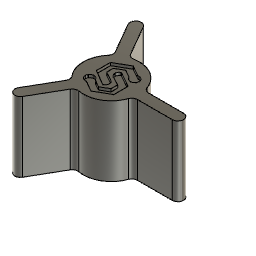
Rotary Cap (Autodesk Fusion 360 design; units mm, degrees)
Autodesk Fusion 360 part; units mm, degrees
note: some values were not read from the file. Set by a fixed rule: which sketch regions a step uses.
sketch "Sketch1" plane through (0, 0, 0) normal (0, 0, 1) x (1, 0, 0)
  circle A0 centre (0, 0) radius 3.15
  line L0 (0, 0) -> (-3.15, 0) construction
  line L1 (-3.15, 0) -> (-3.15, 4) construction
  line L2 (1.4, 2.8218) -> (1.4, -2.8218)
  line L3 (0, 0) -> (7.7021, 0) construction
  line L4 (12.899, 1) -> (4.899, 1)
  line L5 (4.899, -1) -> (12.8981, -1)
  line L6 (12.8981, -1) -> (12.899, 1)
  line L7 (12.899, 1) -> (7.0944, 0) construction
  line L8 (7.0944, 0) -> (12.8981, -1) construction
  arc A1 (4.899, 1) -> (4.899, -1) centre (0, 0) ccw
  line L9 (-7.3155, 10.6708) -> (-3.3155, 3.7426)
  line L10 (-1.5835, 4.7426) -> (-5.583, 11.6701)
  line L11 (-5.583, 11.6701) -> (-7.3155, 10.6708)
  line L12 (-5.5835, -11.6708) -> (-1.5835, -4.7426)
  line L13 (-3.3155, -3.7426) -> (-7.3151, -10.6701)
  line L14 (-7.3151, -10.6701) -> (-5.5835, -11.6708)
  dimension "d1" = 6.3
  dimension "d2" = 4.55
  dimension "d3" = 10
  dimension "d12" = 8
  dimension "d14" = 360
  dimension "d15" = 2
  dimension "d16" = 1
  constraint coincident A0.centre L0.start
  constraint coincident A0 L0.end
  constraint horizontal L0
  constraint tangent A0 L1
  constraint coincident A0 L2.start
  constraint coincident A0 L2.end
  constraint vertical L2
  constraint perpendicular L2 L3
  constraint horizontal L4
  constraint parallel L4 L5
  constraint coincident L3 L7.end
  measures "d1" diameter of A0
  measures "d2" distance of L1 L2
  measures "d3" diameter of A1
  measures "d12" distance of L6 L4.end
  measures "d15" distance of L4 L5
  measures "d16" distance of L3 L4
extrude "Extrude1" add sketch "Sketch1" along normal blind 12.5 contours A0 L2 | L4 L5 L6 A1 | A1 L9 L10 L11 | A1 L12 L13 L14 picked at (2.2591, -0.5149)
sketch "Sketch2" plane through (0, 0, 12.5) normal (0, 0, 1) x (-1, 0, 0)
  arc A0 (-1.4, -2.8218) -> (-1.4, 2.8218) centre (0, 0) ccw
  line L0 (-1.4, -2.8218) -> (-1.4, 2.8218)
  arc A1 (1.5835, 4.7426) -> (-4.899, 1) centre (0, 0) ccw
  line L1 (-4.899, 1) -> (-12.8981, 1)
  line L2 (-12.8981, 1) -> (-12.899, -1)
  line L3 (-12.899, -1) -> (-4.899, -1)
  circle A2 centre (0, 0) radius 3.15
  line L4 (7.3151, 10.6701) -> (5.5835, 11.6708)
  line L5 (5.5835, 11.6708) -> (1.5835, 4.7426)
  arc A3 (-4.899, -1) -> (1.5835, -4.7426) centre (0, 0) ccw
  line L6 (1.5835, -4.7426) -> (5.583, -11.6701)
  line L7 (5.583, -11.6701) -> (7.3155, -10.6708)
  line L8 (7.3155, -10.6708) -> (3.3155, -3.7426)
  arc A4 (3.3155, -3.7426) -> (3.3155, 3.7426) centre (0, 0) ccw
  line L9 (3.3155, 3.7426) -> (7.3151, 10.6701)
  constraint coincident A0.centre A1.centre
  constraint coincident A0.start A2
extrude "Extrude2" add sketch "Sketch2" against normal blind 2 contours A0 L0 A2
fillet "Fillet1" radius 1 12 edges at (4.899, -1, 6.25) (12.8981, -1, 6.25) (12.899, 1, 6.25) (4.899, 1, 6.25) (-1.5835, -4.7426, 6.25) (-3.3155, -3.7426, 6.25) (-3.3155, 3.7426, 6.25) (-1.5835, 4.7426, 6.25) (-5.5835, -11.6708, 6.25) (-7.3151, -10.6701, 6.25) (-7.3155, 10.6708, 6.25) (-5.583, 11.6701, 6.25)
sketch "Sketch3" plane through (0, 0, 12.5) normal (0, 0, 1) x (-1, 0, 0)
  arc A0 (-11.8986, 1) -> (-11.8986, -1) centre (-11.8986, 0) ccw
  line L0 (-11.8986, -1) -> (-5.6569, -1)
  arc A1 (-4.714, -1.6667) -> (-5.6569, -1) centre (-5.6569, -2) ccw
  arc A2 (-4.714, -1.6667) -> (0.9136, -4.9158) centre (0, 0) ccw
  arc A3 (-5.6569, 1) -> (-4.714, 1.6667) centre (-5.6569, 2) ccw
  line L1 (-5.6569, 1) -> (-11.8986, 1)
  spline S0 degree 3 poles (-6.2098, 2.4164) (-5.9078, 2.4164) (-5.6092, 2.3629) (-5.3142, 2.2561) knots 0 0 0 0 1 1 1 1
  spline S1 degree 3 poles (-5.3142, 2.2561) (-5.019, 2.1491) (-4.7505, 1.9819) (-4.509, 1.7542) knots 0 0 0 0 1 1 1 1
  line L2 (-4.509, 1.7542) -> (-5.0946, 1.0362)
  spline S2 degree 3 poles (-5.0946, 1.0362) (-5.2572, 1.171) (-5.4407, 1.2743) (-5.6453, 1.3463) knots 0 0 0 0 1 1 1 1
  spline S3 degree 3 poles (-5.6453, 1.3463) (-5.8497, 1.4185) (-6.0471, 1.4544) (-6.2377, 1.4544) knots 0 0 0 0 1 1 1 1
  spline S4 degree 3 poles (-6.2377, 1.4544) (-6.433, 1.4544) (-6.5781, 1.4219) (-6.6735, 1.3569) knots 0 0 0 0 1 1 1 1
  spline S5 degree 3 poles (-6.6735, 1.3569) (-6.7686, 1.2918) (-6.8164, 1.1989) (-6.8164, 1.078) knots 0 0 0 0 1 1 1 1
  spline S6 degree 3 poles (-6.8164, 1.078) (-6.8164, 0.9897) (-6.7896, 0.9201) (-6.7362, 0.8688) knots 0 0 0 0 1 1 1 1
  spline S7 degree 3 poles (-6.7362, 0.8688) (-6.6827, 0.8178) (-6.6096, 0.7713) (-6.5165, 0.7295) knots 0 0 0 0 1 1 1 1
  spline S8 degree 3 poles (-6.5165, 0.7295) (-6.4236, 0.6876) (-6.3121, 0.6413) (-6.182, 0.59) knots 0 0 0 0 1 1 1 1
  line L3 (-6.182, 0.59) -> (-5.6034, 0.3461)
  spline S9 degree 3 poles (-5.6034, 0.3461) (-5.4407, 0.281) (-5.2898, 0.1927) (-5.1503, 0.0812) knots 0 0 0 0 1 1 1 1
  spline S10 degree 3 poles (-5.1503, 0.0812) (-5.0109, -0.0304) (-4.8982, -0.1686) (-4.8122, -0.3336) knots 0 0 0 0 1 1 1 1
  spline S11 degree 3 poles (-4.8122, -0.3336) (-4.7262, -0.4985) (-4.6833, -0.6902) (-4.6833, -0.9087) knots 0 0 0 0 1 1 1 1
  spline S12 degree 3 poles (-4.6833, -0.9087) (-4.6833, -1.1642) (-4.7541, -1.3954) (-4.896, -1.6022) knots 0 0 0 0 1 1 1 1
  spline S13 degree 3 poles (-4.896, -1.6022) (-5.0376, -1.809) (-5.2327, -1.9751) (-5.4814, -2.1007) knots 0 0 0 0 1 1 1 1
  spline S14 degree 3 poles (-5.4814, -2.1007) (-5.7299, -2.2261) (-6.0169, -2.2889) (-6.3423, -2.2889) knots 0 0 0 0 1 1 1 1
  spline S15 degree 3 poles (-6.3423, -2.2889) (-6.6164, -2.2889) (-6.8826, -2.24) (-7.1404, -2.1425) knots 0 0 0 0 1 1 1 1
  spline S16 degree 3 poles (-7.1404, -2.1425) (-7.3984, -2.0449) (-7.625, -1.9032) (-7.8201, -1.7173) knots 0 0 0 0 1 1 1 1
  line L4 (-7.8201, -1.7173) -> (-7.2416, -0.9923)
  spline S17 degree 3 poles (-7.2416, -0.9923) (-7.0882, -1.1039) (-6.936, -1.1875) (-6.785, -1.2432) knots 0 0 0 0 1 1 1 1
  spline S18 degree 3 poles (-6.785, -1.2432) (-6.6339, -1.299) (-6.4863, -1.3269) (-6.3423, -1.3269) knots 0 0 0 0 1 1 1 1
  spline S19 degree 3 poles (-6.3423, -1.3269) (-6.1797, -1.3269) (-6.0506, -1.2966) (-5.9555, -1.2363) knots 0 0 0 0 1 1 1 1
  spline S20 degree 3 poles (-5.9555, -1.2363) (-5.8601, -1.1758) (-5.8125, -1.0875) (-5.8125, -0.9714) knots 0 0 0 0 1 1 1 1
  spline S21 degree 3 poles (-5.8125, -0.9714) (-5.8125, -0.8924) (-5.8404, -0.825) (-5.8962, -0.7692) knots 0 0 0 0 1 1 1 1
  spline S22 degree 3 poles (-5.8962, -0.7692) (-5.952, -0.7135) (-6.0321, -0.6647) (-6.1367, -0.6229) knots 0 0 0 0 1 1 1 1
  spline S23 degree 3 poles (-6.1367, -0.6229) (-6.2413, -0.581) (-6.3608, -0.5323) (-6.4957, -0.4764) knots 0 0 0 0 1 1 1 1
  line L5 (-6.4957, -0.4764) -> (-7.0602, -0.2534)
  spline S24 degree 3 poles (-7.0602, -0.2534) (-7.2461, -0.179) (-7.4053, -0.0849) (-7.5378, 0.0289) knots 0 0 0 0 1 1 1 1
  spline S25 degree 3 poles (-7.5378, 0.0289) (-7.6702, 0.1428) (-7.7723, 0.2776) (-7.8445, 0.4331) knots 0 0 0 0 1 1 1 1
  spline S26 degree 3 poles (-7.8445, 0.4331) (-7.9165, 0.589) (-7.9526, 0.7737) (-7.9526, 0.9873) knots 0 0 0 0 1 1 1 1
  spline S27 degree 3 poles (-7.9526, 0.9873) (-7.9526, 1.243) (-7.8852, 1.4788) (-7.7504, 1.6949) knots 0 0 0 0 1 1 1 1
  spline S28 degree 3 poles (-7.7504, 1.6949) (-7.6156, 1.911) (-7.4181, 2.0853) (-7.1579, 2.2178) knots 0 0 0 0 1 1 1 1
  spline S29 degree 3 poles (-7.1579, 2.2178) (-6.8975, 2.3502) (-6.5816, 2.4164) (-6.2098, 2.4164) knots 0 0 0 0 1 1 1 1
  spline S30 degree 3 poles (-10.3713, 1.4544) (-10.5666, 1.4544) (-10.735, 1.3976) (-10.8767, 1.2836) knots 0 0 0 0 1 1 1 1
  spline S31 degree 3 poles (-10.8767, 1.2836) (-11.0184, 1.1698) (-11.1265, 1.0072) (-11.2009, 0.7957) knots 0 0 0 0 1 1 1 1
  spline S32 degree 3 poles (-11.2009, 0.7957) (-11.2752, 0.5842) (-11.3124, 0.3345) (-11.3124, 0.0463) knots 0 0 0 0 1 1 1 1
  spline S33 degree 3 poles (-11.3124, 0.0463) (-11.3124, -0.2465) (-11.2752, -0.4939) (-11.2009, -0.6961) knots 0 0 0 0 1 1 1 1
  spline S34 degree 3 poles (-11.2009, -0.6961) (-11.1265, -0.8982) (-11.0184, -1.0539) (-10.8767, -1.1632) knots 0 0 0 0 1 1 1 1
  spline S35 degree 3 poles (-10.8767, -1.1632) (-10.735, -1.2722) (-10.5666, -1.3269) (-10.3713, -1.3269) knots 0 0 0 0 1 1 1 1
  spline S36 degree 3 poles (-10.3713, -1.3269) (-10.1762, -1.3269) (-10.0077, -1.2722) (-9.8659, -1.1632) knots 0 0 0 0 1 1 1 1
  spline S37 degree 3 poles (-9.8659, -1.1632) (-9.7242, -1.0539) (-9.6162, -0.8982) (-9.5419, -0.6961) knots 0 0 0 0 1 1 1 1
  spline S38 degree 3 poles (-9.5419, -0.6961) (-9.4675, -0.4939) (-9.4303, -0.2465) (-9.4303, 0.0463) knots 0 0 0 0 1 1 1 1
  spline S39 degree 3 poles (-9.4303, 0.0463) (-9.4303, 0.3345) (-9.4675, 0.5842) (-9.5419, 0.7957) knots 0 0 0 0 1 1 1 1
  spline S40 degree 3 poles (-9.5419, 0.7957) (-9.6162, 1.0072) (-9.7242, 1.1698) (-9.8659, 1.2836) knots 0 0 0 0 1 1 1 1
  spline S41 degree 3 poles (-9.8659, 1.2836) (-10.0077, 1.3976) (-10.1762, 1.4544) (-10.3713, 1.4544) knots 0 0 0 0 1 1 1 1
  spline S42 degree 3 poles (-10.3713, 2.4164) (-9.9577, 2.4164) (-9.5941, 2.3223) (-9.2804, 2.1341) knots 0 0 0 0 1 1 1 1
  spline S43 degree 3 poles (-9.2804, 2.1341) (-8.9668, 1.9458) (-8.7228, 1.674) (-8.5486, 1.3185) knots 0 0 0 0 1 1 1 1
  spline S44 degree 3 poles (-8.5486, 1.3185) (-8.3743, 0.963) (-8.287, 0.5389) (-8.287, 0.0463) knots 0 0 0 0 1 1 1 1
  spline S45 degree 3 poles (-8.287, 0.0463) (-8.287, -0.451) (-8.3743, -0.8727) (-8.5486, -1.2188) knots 0 0 0 0 1 1 1 1
  spline S46 degree 3 poles (-8.5486, -1.2188) (-8.7228, -1.565) (-8.9668, -1.8299) (-9.2804, -2.0135) knots 0 0 0 0 1 1 1 1
  spline S47 degree 3 poles (-9.2804, -2.0135) (-9.5941, -2.1971) (-9.9577, -2.2889) (-10.3713, -2.2889) knots 0 0 0 0 1 1 1 1
  spline S48 degree 3 poles (-10.3713, -2.2889) (-10.7849, -2.2889) (-11.1486, -2.1971) (-11.4623, -2.0135) knots 0 0 0 0 1 1 1 1
  spline S49 degree 3 poles (-11.4623, -2.0135) (-11.7759, -1.8299) (-12.0199, -1.565) (-12.1943, -1.2188) knots 0 0 0 0 1 1 1 1
  spline S50 degree 3 poles (-12.1943, -1.2188) (-12.3685, -0.8727) (-12.4556, -0.451) (-12.4556, 0.0463) knots 0 0 0 0 1 1 1 1
  spline S51 degree 3 poles (-12.4556, 0.0463) (-12.4556, 0.5389) (-12.3685, 0.963) (-12.1943, 1.3185) knots 0 0 0 0 1 1 1 1
  spline S52 degree 3 poles (-12.1943, 1.3185) (-12.0199, 1.674) (-11.7759, 1.9458) (-11.4623, 2.1341) knots 0 0 0 0 1 1 1 1
  spline S53 degree 3 poles (-11.4623, 2.1341) (-11.1486, 2.3223) (-10.7849, 2.4164) (-10.3713, 2.4164) knots 0 0 0 0 1 1 1 1
  line L6 (-17.4953, 1.4404) -> (-17.6278, 1.4404)
  spline S54 degree 3 poles (-17.6278, 1.4404) (-17.8647, 1.4404) (-18.0763, 1.3986) (-18.2621, 1.315) knots 0 0 0 0 1 1 1 1
  spline S55 degree 3 poles (-18.2621, 1.315) (-18.448, 1.2314) (-18.5943, 1.0885) (-18.7013, 0.8862) knots 0 0 0 0 1 1 1 1
  spline S56 degree 3 poles (-18.7013, 0.8862) (-18.8081, 0.6841) (-18.8616, 0.4043) (-18.8616, 0.0462) knots 0 0 0 0 1 1 1 1
  spline S57 degree 3 poles (-18.8616, 0.0462) (-18.8616, -0.3115) (-18.8081, -0.588) (-18.7013, -0.7832) knots 0 0 0 0 1 1 1 1
  spline S58 degree 3 poles (-18.7013, -0.7832) (-18.5943, -0.9783) (-18.448, -1.1154) (-18.2621, -1.1944) knots 0 0 0 0 1 1 1 1
  spline S59 degree 3 poles (-18.2621, -1.1944) (-18.0763, -1.2735) (-17.8647, -1.313) (-17.6278, -1.313) knots 0 0 0 0 1 1 1 1
  line L7 (-17.6278, -1.313) -> (-17.4953, -1.313)
  line L8 (-17.4953, -1.313) -> (-17.4953, 1.4404)
  line L9 (-16.38, 2.3327) -> (-16.38, -2.2052)
  line L10 (-16.38, -2.2052) -> (-17.6975, -2.2052)
  spline S60 degree 3 poles (-17.6975, -2.2052) (-18.1576, -2.2052) (-18.5607, -2.1274) (-18.907, -1.9718) knots 0 0 0 0 1 1 1 1
  spline S61 degree 3 poles (-18.907, -1.9718) (-19.253, -1.816) (-19.5214, -1.5732) (-19.7121, -1.2432) knots 0 0 0 0 1 1 1 1
  spline S62 degree 3 poles (-19.7121, -1.2432) (-19.9025, -0.9132) (-19.9978, -0.4835) (-19.9978, 0.0462) knots 0 0 0 0 1 1 1 1
  spline S63 degree 3 poles (-19.9978, 0.0462) (-19.9978, 0.5715) (-19.9025, 1.0026) (-19.7121, 1.3394) knots 0 0 0 0 1 1 1 1
  spline S64 degree 3 poles (-19.7121, 1.3394) (-19.5214, 1.6764) (-19.2578, 1.9261) (-18.9209, 2.0887) knots 0 0 0 0 1 1 1 1
  spline S65 degree 3 poles (-18.9209, 2.0887) (-18.5839, 2.2514) (-18.197, 2.3327) (-17.7602, 2.3327) knots 0 0 0 0 1 1 1 1
  line L11 (-17.7602, 2.3327) -> (-16.38, 2.3327)
  line L12 (-20.5074, 2.3327) -> (-20.5074, -2.2052)
  line L13 (-20.5074, -2.2052) -> (-23.4002, -2.2052)
  line L14 (-23.4002, -2.2052) -> (-23.4002, -1.2711)
  line L15 (-23.4002, -1.2711) -> (-21.6227, -1.2711)
  line L16 (-21.6227, -1.2711) -> (-21.6227, -0.4625)
  line L17 (-21.6227, -0.4625) -> (-23.1354, -0.4625)
  line L18 (-23.1354, -0.4625) -> (-23.1354, 0.4715)
  line L19 (-23.1354, 0.4715) -> (-21.6227, 0.4715)
  line L20 (-21.6227, 0.4715) -> (-21.6227, 1.3986)
  line L21 (-21.6227, 1.3986) -> (-23.47, 1.3986)
  line L22 (-23.47, 1.3986) -> (-23.47, 2.3327)
  line L23 (-23.47, 2.3327) -> (-20.5074, 2.3327)
  line L24 (-25.1917, -1.32) -> (-25.6727, -1.32)
  spline S66 degree 3 poles (-25.6727, -1.32) (-25.9236, -1.32) (-26.1152, -1.2804) (-26.2477, -1.2015) knots 0 0 0 0 1 1 1 1
  spline S67 degree 3 poles (-26.2477, -1.2015) (-26.3801, -1.1224) (-26.4464, -0.9759) (-26.4464, -0.7623) knots 0 0 0 0 1 1 1 1
  spline S68 degree 3 poles (-26.4464, -0.7623) (-26.4464, -0.5531) (-26.3801, -0.3951) (-26.2477, -0.2882) knots 0 0 0 0 1 1 1 1
  spline S69 degree 3 poles (-26.2477, -0.2882) (-26.1152, -0.1813) (-25.9236, -0.128) (-25.6727, -0.128) knots 0 0 0 0 1 1 1 1
  line L25 (-25.6727, -0.128) -> (-25.1917, -0.128)
  line L26 (-25.1917, -0.128) -> (-25.1917, -1.32)
  line L27 (-27.7709, 2.3327) -> (-26.7633, 0.5394)
  spline S70 degree 3 poles (-26.7633, 0.5394) (-26.9762, 0.4339) (-27.1545, 0.2898) (-27.2934, 0.1021) knots 0 0 0 0 1 1 1 1
  spline S71 degree 3 poles (-27.2934, 0.1021) (-27.4583, -0.121) (-27.5409, -0.4091) (-27.5409, -0.7623) knots 0 0 0 0 1 1 1 1
  spline S72 degree 3 poles (-27.5409, -0.7623) (-27.5409, -1.134) (-27.4583, -1.4246) (-27.2934, -1.6336) knots 0 0 0 0 1 1 1 1
  spline S73 degree 3 poles (-27.2934, -1.6336) (-27.1283, -1.8427) (-26.9111, -1.9902) (-26.6416, -2.0763) knots 0 0 0 0 1 1 1 1
  spline S74 degree 3 poles (-26.6416, -2.0763) (-26.372, -2.1623) (-26.0769, -2.2052) (-25.7564, -2.2052) knots 0 0 0 0 1 1 1 1
  line L28 (-25.7564, -2.2052) -> (-24.0764, -2.2052)
  line L29 (-24.0764, -2.2052) -> (-24.0764, 2.3327)
  line L30 (-24.0764, 2.3327) -> (-25.1917, 2.3327)
  line L31 (-25.1917, 2.3327) -> (-25.1917, 0.7574)
  line L32 (-25.1917, 0.7574) -> (-25.7071, 0.7574)
  line L33 (-25.7071, 0.7574) -> (-26.5301, 2.3327)
  line L34 (-26.5301, 2.3327) -> (-27.7709, 2.3327)
  line L35 (-28.2029, 2.3327) -> (-28.2029, -2.2052)
  line L36 (-28.2029, -2.2052) -> (-31.0958, -2.2052)
  line L37 (-31.0958, -2.2052) -> (-31.0958, -1.2711)
  line L38 (-31.0958, -1.2711) -> (-29.3182, -1.2711)
  line L39 (-29.3182, -1.2711) -> (-29.3182, -0.4625)
  line L40 (-29.3182, -0.4625) -> (-30.8309, -0.4625)
  line L41 (-30.8309, -0.4625) -> (-30.8309, 0.4715)
  line L42 (-30.8309, 0.4715) -> (-29.3182, 0.4715)
  line L43 (-29.3182, 0.4715) -> (-29.3182, 1.3986)
  line L44 (-29.3182, 1.3986) -> (-31.1655, 1.3986)
  line L45 (-31.1655, 1.3986) -> (-31.1655, 2.3327)
  line L46 (-31.1655, 2.3327) -> (-28.2029, 2.3327)
  line L47 (-32.8176, 1.4404) -> (-32.95, 1.4404)
  spline S75 degree 3 poles (-32.95, 1.4404) (-33.187, 1.4404) (-33.3985, 1.3986) (-33.5843, 1.315) knots 0 0 0 0 1 1 1 1
  spline S76 degree 3 poles (-33.5843, 1.315) (-33.7702, 1.2314) (-33.9166, 1.0885) (-34.0235, 0.8862) knots 0 0 0 0 1 1 1 1
  spline S77 degree 3 poles (-34.0235, 0.8862) (-34.1303, 0.6841) (-34.1838, 0.4043) (-34.1838, 0.0462) knots 0 0 0 0 1 1 1 1
  spline S78 degree 3 poles (-34.1838, 0.0462) (-34.1838, -0.3115) (-34.1303, -0.588) (-34.0235, -0.7832) knots 0 0 0 0 1 1 1 1
  spline S79 degree 3 poles (-34.0235, -0.7832) (-33.9166, -0.9783) (-33.7702, -1.1154) (-33.5843, -1.1944) knots 0 0 0 0 1 1 1 1
  spline S80 degree 3 poles (-33.5843, -1.1944) (-33.3985, -1.2735) (-33.187, -1.313) (-32.95, -1.313) knots 0 0 0 0 1 1 1 1
  line L48 (-32.95, -1.313) -> (-32.8176, -1.313)
  line L49 (-32.8176, -1.313) -> (-32.8176, 1.4404)
  line L50 (-31.7023, 2.3327) -> (-31.7023, -2.2052)
  line L51 (-31.7023, -2.2052) -> (-33.0197, -2.2052)
  spline S81 degree 3 poles (-33.0197, -2.2052) (-33.4798, -2.2052) (-33.8829, -2.1274) (-34.2292, -1.9718) knots 0 0 0 0 1 1 1 1
  spline S82 degree 3 poles (-34.2292, -1.9718) (-34.5753, -1.816) (-34.8436, -1.5732) (-35.0343, -1.2432) knots 0 0 0 0 1 1 1 1
  spline S83 degree 3 poles (-35.0343, -1.2432) (-35.2248, -0.9132) (-35.32, -0.4835) (-35.32, 0.0462) knots 0 0 0 0 1 1 1 1
  spline S84 degree 3 poles (-35.32, 0.0462) (-35.32, 0.5715) (-35.2248, 1.0026) (-35.0343, 1.3394) knots 0 0 0 0 1 1 1 1
  spline S85 degree 3 poles (-35.0343, 1.3394) (-34.8436, 1.6764) (-34.5801, 1.9261) (-34.2431, 2.0887) knots 0 0 0 0 1 1 1 1
  spline S86 degree 3 poles (-34.2431, 2.0887) (-33.9061, 2.2514) (-33.5193, 2.3327) (-33.0825, 2.3327) knots 0 0 0 0 1 1 1 1
  line L52 (-33.0825, 2.3327) -> (-31.7023, 2.3327)
  line L53 (-14.6781, 1.2454) -> (-14.052, 0.6192)
  line L54 (-14.052, 0.6192) -> (-14.052, -2.2052)
  line L55 (-14.052, -2.2052) -> (-12.9366, -2.2052)
  line L56 (-12.9366, -2.2052) -> (-12.9366, 1.1617)
  line L57 (-12.9366, 1.1617) -> (-14.0947, 2.3197)
  line L58 (-14.0947, 2.3197) -> (-15.8425, 2.3197)
  line L59 (-15.8425, 2.3197) -> (-15.8425, 1.2454)
  line L60 (-15.8425, 1.2454) -> (-14.6781, 1.2454)
  line L61 (-2.2394, -2.7135) -> (-2.2375, -2.7135)
  spline S87 degree 3 poles (-2.2375, -2.7135) (-2.0945, -2.7132) (-1.9536, -2.7479) (-1.8297, -2.8194) knots 0 0 0 0 1 1 1 1
  line L62 (-1.8297, -2.8194) -> (-0.1005, -3.8178)
  line L63 (-0.1005, -3.8178) -> (2.4914, -2.3226)
  line L64 (2.4914, -2.3226) -> (2.4914, 0.1947)
  line L65 (2.4914, 0.1947) -> (-0.234, 1.7682)
  line L66 (-0.234, 1.7682) -> (-0.2972, 1.7352)
  spline S88 degree 3 poles (-0.2972, 1.7352) (-0.5334, 1.613) (-0.7079, 1.3532) (-0.7117, 1.0874) knots 0 0 0 0 1 1 1 1
  spline S89 degree 3 poles (-0.7117, 1.0874) (-0.7155, 0.8215) (-0.5476, 0.5233) (-0.3152, 0.3946) knots 0 0 0 0 1 1 1 1
  line L67 (-0.3152, 0.3946) -> (1.3304, -0.4892)
  line L68 (1.3304, -0.4892) -> (1.3304, -1.6688)
  line L69 (1.3304, -1.6688) -> (-0.0948, -2.4992)
  line L70 (-0.0948, -2.4992) -> (-1.2895, -1.8007)
  spline S90 degree 3 poles (-1.2895, -1.8007) (-1.4025, -1.7347) (-1.4943, -1.639) (-1.5608, -1.5262) knots 0 0 0 0 1 1 1 1
  spline S91 degree 3 poles (-1.5608, -1.5262) (-1.6978, -1.2941) (-1.9504, -1.1383) (-2.2394, -1.1383) knots 0 0 0 0 1 1 1 1
  spline S92 degree 3 poles (-2.2394, -1.1383) (-2.5025, -1.1383) (-2.7353, -1.2674) (-2.8784, -1.4657) knots 0 0 0 0 1 1 1 1
  spline S93 degree 3 poles (-2.8784, -1.4657) (-2.8921, -1.484) (-2.905, -1.5032) (-2.9167, -1.5235) knots 0 0 0 0 1 1 1 1
  spline S94 degree 3 poles (-2.9167, -1.5235) (-2.9182, -1.5261) (-2.9195, -1.5287) (-2.921, -1.5314) knots 0 0 0 0 1 1 1 1
  spline S95 degree 3 poles (-2.921, -1.5314) (-2.9883, -1.6474) (-3.027, -1.7821) (-3.027, -1.9259) knots 0 0 0 0 1 1 1 1
  spline S96 degree 3 poles (-3.027, -1.9259) (-3.027, -2.3609) (-2.6744, -2.7135) (-2.2394, -2.7135) knots 0 0 0 0 1 1 1 1
  spline S97 degree 3 poles (0.0025, -1.7208) (0.2386, -1.5986) (0.4131, -1.3388) (0.417, -1.073) knots 0 0 0 0 1 1 1 1
  spline S98 degree 3 poles (0.417, -1.073) (0.4207, -0.8071) (0.2528, -0.5089) (0.0204, -0.3802) knots 0 0 0 0 1 1 1 1
  line L71 (0.0204, -0.3802) -> (-1.6252, 0.5036)
  line L72 (-1.6252, 0.5036) -> (-1.6252, 1.6832)
  line L73 (-1.6252, 1.6832) -> (-0.1999, 2.5136)
  line L74 (-0.1999, 2.5136) -> (0.9947, 1.8151)
  spline S99 degree 3 poles (0.9947, 1.8151) (1.1077, 1.7491) (1.1996, 1.6534) (1.2661, 1.5407) knots 0 0 0 0 1 1 1 1
  spline S100 degree 3 poles (1.2661, 1.5407) (1.4031, 1.3085) (1.6556, 1.1528) (1.9447, 1.1528) knots 0 0 0 0 1 1 1 1
  spline S101 degree 3 poles (1.9447, 1.1528) (2.2078, 1.1528) (2.4405, 1.2819) (2.5836, 1.4801) knots 0 0 0 0 1 1 1 1
  spline S102 degree 3 poles (2.5836, 1.4801) (2.5973, 1.4984) (2.6102, 1.5176) (2.6219, 1.5379) knots 0 0 0 0 1 1 1 1
  spline S103 degree 3 poles (2.6219, 1.5379) (2.6234, 1.5405) (2.6247, 1.5432) (2.6262, 1.5457) knots 0 0 0 0 1 1 1 1
  spline S104 degree 3 poles (2.6262, 1.5457) (2.6935, 1.6618) (2.7322, 1.7965) (2.7322, 1.9403) knots 0 0 0 0 1 1 1 1
  spline S105 degree 3 poles (2.7322, 1.9403) (2.7322, 2.3753) (2.3796, 2.7279) (1.9447, 2.7279) knots 0 0 0 0 1 1 1 1
  line L75 (1.9447, 2.7279) -> (1.9428, 2.7279)
  spline S106 degree 3 poles (1.9428, 2.7279) (1.7997, 2.7276) (1.6588, 2.7623) (1.5349, 2.8338) knots 0 0 0 0 1 1 1 1
  line L76 (1.5349, 2.8338) -> (-0.1943, 3.8322)
  line L77 (-0.1943, 3.8322) -> (-2.7861, 2.337)
  line L78 (-2.7861, 2.337) -> (-2.7861, -0.1803)
  line L79 (-2.7861, -0.1803) -> (-0.0608, -1.7538)
  line L80 (-0.0608, -1.7538) -> (0.0025, -1.7208)
  line L81 (1.9624, -5.399) -> (5.0833, -10.8044)
  line L82 (6.8153, -9.8044) -> (3.6945, -4.399)
  line L83 (3.6945, 4.399) -> (6.8153, 9.8044)
  line L84 (5.0833, 10.8044) -> (1.9624, 5.399)
  arc A4 (1.9624, -5.399) -> (0.9136, -4.9158) centre (1.0964, -5.899) ccw
  arc A5 (3.8004, -3.2491) -> (3.6945, -4.399) centre (4.5605, -3.899) ccw
  arc A6 (3.8004, -3.2491) -> (3.8004, 3.2491) centre (0, 0) ccw
  arc A7 (3.6945, 4.399) -> (3.8004, 3.2491) centre (4.5605, 3.899) ccw
  arc A8 (0.9136, 4.9158) -> (1.9624, 5.399) centre (1.0964, 5.899) ccw
  arc A9 (0.9136, 4.9158) -> (-4.714, 1.6667) centre (0, 0) ccw
  arc A10 (5.0833, -10.8044) -> (6.8153, -9.8044) centre (5.9493, -10.3044) ccw
  arc A11 (6.8153, 9.8044) -> (5.0833, 10.8044) centre (5.9493, 10.3044) ccw
extrude "Extrude3" cut sketch "Sketch3" against normal blind 0.5 contours S87 L62 L63 L64 L65 L66 S88 S89 L67 L68 L69 L70 S90 S91 S92 S93 S94 S95 S96 | S97 S98 L71 L72 L73 L74 S99 S100 S101 S102 S103 S104 S105 S106 L76 L77 L78 L79 L80
chamfer "Chamfer1" distance 1 angle 45 2 edges at (1.4, 0, 0) (-3.15, 0, 0)
